Autodesk Fusion 360 part; units mm, degrees
(part 3 of 14)
  line L362 (718.6407, 200.025) -> (707.6422, 200.025)
  line L363 (707.6422, 200.025) -> (702.1429, 190.5)
  line L364 (702.1429, 190.5) -> (707.6422, 180.975)
  line L365 (707.6422, 180.975) -> (718.6407, 180.975)
  line L366 (724.1399, 190.5) -> (718.6407, 200.025)
  line L367 (718.6407, 180.975) -> (724.1399, 190.5)
  line L368 (737.8881, 211.1375) -> (726.8896, 211.1375)
  line L369 (726.8896, 211.1375) -> (721.3903, 201.6125)
  line L370 (721.3903, 201.6125) -> (726.8896, 192.0875)
  line L371 (726.8896, 192.0875) -> (737.8881, 192.0875)
  line L372 (743.3874, 201.6125) -> (737.8881, 211.1375)
  line L373 (737.8881, 192.0875) -> (743.3874, 201.6125)
  line L374 (757.1355, 222.25) -> (746.137, 222.25)
  line L375 (746.137, 222.25) -> (740.6377, 212.725)
  line L376 (740.6377, 212.725) -> (746.137, 203.2)
  line L377 (746.137, 203.2) -> (757.1355, 203.2)
  line L378 (762.6348, 212.725) -> (757.1355, 222.25)
  line L379 (757.1355, 203.2) -> (762.6348, 212.725)
  line L380 (-397.7094, -422.275) -> (-408.7079, -422.275)
  line L381 (-408.7079, -422.275) -> (-414.2072, -431.8)
  line L382 (-414.2072, -431.8) -> (-408.7079, -441.325)
  line L383 (-408.7079, -441.325) -> (-397.7094, -441.325)
  line L384 (-392.2101, -431.8) -> (-397.7094, -422.275)
  line L385 (-397.7094, -441.325) -> (-392.2101, -431.8)
  line L386 (-378.462, -411.1625) -> (-389.4605, -411.1625)
  line L387 (-389.4605, -411.1625) -> (-394.9597, -420.6875)
  line L388 (-394.9597, -420.6875) -> (-389.4605, -430.2125)
  line L389 (-389.4605, -430.2125) -> (-378.462, -430.2125)
  line L390 (-372.9627, -420.6875) -> (-378.462, -411.1625)
  line L391 (-378.462, -430.2125) -> (-372.9627, -420.6875)
  line L392 (-359.2145, -400.05) -> (-370.2131, -400.05)
  line L393 (-370.2131, -400.05) -> (-375.7123, -409.575)
  line L394 (-375.7123, -409.575) -> (-370.2131, -419.1)
  line L395 (-370.2131, -419.1) -> (-359.2145, -419.1)
  line L396 (-353.7153, -409.575) -> (-359.2145, -400.05)
  line L397 (-359.2145, -419.1) -> (-353.7153, -409.575)
  line L398 (-339.9671, -388.9375) -> (-350.9657, -388.9375)
  line L399 (-350.9657, -388.9375) -> (-356.4649, -398.4625)
  line L400 (-356.4649, -398.4625) -> (-350.9657, -407.9875)
  line L401 (-350.9657, -407.9875) -> (-339.9671, -407.9875)
  line L402 (-334.4679, -398.4625) -> (-339.9671, -388.9375)
  line L403 (-339.9671, -407.9875) -> (-334.4679, -398.4625)
  line L404 (-320.7197, -377.825) -> (-331.7182, -377.825)
  line L405 (-331.7182, -377.825) -> (-337.2175, -387.35)
  line L406 (-337.2175, -387.35) -> (-331.7182, -396.875)
  line L407 (-331.7182, -396.875) -> (-320.7197, -396.875)
  line L408 (-315.2205, -387.35) -> (-320.7197, -377.825)
  line L409 (-320.7197, -396.875) -> (-315.2205, -387.35)
  line L410 (-301.4723, -366.7125) -> (-312.4708, -366.7125)
  line L411 (-312.4708, -366.7125) -> (-317.9701, -376.2375)
  line L412 (-317.9701, -376.2375) -> (-312.4708, -385.7625)
  line L413 (-312.4708, -385.7625) -> (-301.4723, -385.7625)
  line L414 (-295.973, -376.2375) -> (-301.4723, -366.7125)
  line L415 (-301.4723, -385.7625) -> (-295.973, -376.2375)
  line L416 (-282.2249, -355.6) -> (-293.2234, -355.6)
  line L417 (-293.2234, -355.6) -> (-298.7227, -365.125)
  line L418 (-298.7227, -365.125) -> (-293.2234, -374.65)
  line L419 (-293.2234, -374.65) -> (-282.2249, -374.65)
  line L420 (-276.7256, -365.125) -> (-282.2249, -355.6)
  line L421 (-282.2249, -374.65) -> (-276.7256, -365.125)
  line L422 (-262.9775, -344.4875) -> (-273.976, -344.4875)
  line L423 (-273.976, -344.4875) -> (-279.4753, -354.0125)
  line L424 (-279.4753, -354.0125) -> (-273.976, -363.5375)
  line L425 (-273.976, -363.5375) -> (-262.9775, -363.5375)
  line L426 (-257.4782, -354.0125) -> (-262.9775, -344.4875)
  line L427 (-262.9775, -363.5375) -> (-257.4782, -354.0125)
  line L428 (-243.7301, -333.375) -> (-254.7286, -333.375)
  line L429 (-254.7286, -333.375) -> (-260.2278, -342.9)
  line L430 (-260.2278, -342.9) -> (-254.7286, -352.425)
  line L431 (-254.7286, -352.425) -> (-243.7301, -352.425)
  line L432 (-238.2308, -342.9) -> (-243.7301, -333.375)
  line L433 (-243.7301, -352.425) -> (-238.2308, -342.9)
  line L434 (-224.4826, -322.2625) -> (-235.4812, -322.2625)
  line L435 (-235.4812, -322.2625) -> (-240.9804, -331.7875)
  line L436 (-240.9804, -331.7875) -> (-235.4812, -341.3125)
  line L437 (-235.4812, -341.3125) -> (-224.4826, -341.3125)
  line L438 (-218.9834, -331.7875) -> (-224.4826, -322.2625)
  line L439 (-224.4826, -341.3125) -> (-218.9834, -331.7875)
  line L440 (-205.2352, -311.15) -> (-216.2337, -311.15)
  line L441 (-216.2337, -311.15) -> (-221.733, -320.675)
  line L442 (-221.733, -320.675) -> (-216.2337, -330.2)
  line L443 (-216.2337, -330.2) -> (-205.2352, -330.2)
  line L444 (-199.736, -320.675) -> (-205.2352, -311.15)
  line L445 (-205.2352, -330.2) -> (-199.736, -320.675)
  line L446 (-185.9878, -300.0375) -> (-196.9863, -300.0375)
  line L447 (-196.9863, -300.0375) -> (-202.4856, -309.5625)
  line L448 (-202.4856, -309.5625) -> (-196.9863, -319.0875)
  line L449 (-196.9863, -319.0875) -> (-185.9878, -319.0875)
  line L450 (-180.4886, -309.5625) -> (-185.9878, -300.0375)
  line L451 (-185.9878, -319.0875) -> (-180.4886, -309.5625)
  line L452 (-166.7404, -288.925) -> (-177.7389, -288.925)
  line L453 (-177.7389, -288.925) -> (-183.2382, -298.45)
  line L454 (-183.2382, -298.45) -> (-177.7389, -307.975)
  line L455 (-177.7389, -307.975) -> (-166.7404, -307.975)
  line L456 (-161.2411, -298.45) -> (-166.7404, -288.925)
  line L457 (-166.7404, -307.975) -> (-161.2411, -298.45)
  line L458 (-147.493, -277.8125) -> (-158.4915, -277.8125)
  line L459 (-158.4915, -277.8125) -> (-163.9908, -287.3375)
  line L460 (-163.9908, -287.3375) -> (-158.4915, -296.8625)
  line L461 (-158.4915, -296.8625) -> (-147.493, -296.8625)
  line L462 (-141.9937, -287.3375) -> (-147.493, -277.8125)
  line L463 (-147.493, -296.8625) -> (-141.9937, -287.3375)
  line L464 (-128.2456, -266.7) -> (-139.2441, -266.7)
  line L465 (-139.2441, -266.7) -> (-144.7434, -276.225)
  line L466 (-144.7434, -276.225) -> (-139.2441, -285.75)
  line L467 (-139.2441, -285.75) -> (-128.2456, -285.75)
  line L468 (-122.7463, -276.225) -> (-128.2456, -266.7)
  line L469 (-128.2456, -285.75) -> (-122.7463, -276.225)
  line L470 (-108.9982, -255.5875) -> (-119.9967, -255.5875)
  line L471 (-119.9967, -255.5875) -> (-125.4959, -265.1125)
  line L472 (-125.4959, -265.1125) -> (-119.9967, -274.6375)
  line L473 (-119.9967, -274.6375) -> (-108.9982, -274.6375)
  line L474 (-103.4989, -265.1125) -> (-108.9982, -255.5875)
  line L475 (-108.9982, -274.6375) -> (-103.4989, -265.1125)
  line L476 (-89.7507, -244.475) -> (-100.7493, -244.475)
  line L477 (-100.7493, -244.475) -> (-106.2485, -254)
  line L478 (-106.2485, -254) -> (-100.7493, -263.525)
  line L479 (-100.7493, -263.525) -> (-89.7507, -263.525)
  line L480 (-84.2515, -254) -> (-89.7507, -244.475)
  line L481 (-89.7507, -263.525) -> (-84.2515, -254)
  line L482 (-70.5033, -233.3625) -> (-81.5018, -233.3625)
  line L483 (-81.5018, -233.3625) -> (-87.0011, -242.8875)
  line L484 (-87.0011, -242.8875) -> (-81.5018, -252.4125)
  line L485 (-81.5018, -252.4125) -> (-70.5033, -252.4125)
  line L486 (-65.0041, -242.8875) -> (-70.5033, -233.3625)
  line L487 (-70.5033, -252.4125) -> (-65.0041, -242.8875)
  line L488 (-51.2559, -222.25) -> (-62.2544, -222.25)
  line L489 (-62.2544, -222.25) -> (-67.7537, -231.775)
  line L490 (-67.7537, -231.775) -> (-62.2544, -241.3)
  line L491 (-62.2544, -241.3) -> (-51.2559, -241.3)
  line L492 (-45.7566, -231.775) -> (-51.2559, -222.25)
  line L493 (-51.2559, -241.3) -> (-45.7566, -231.775)
  line L494 (-32.0085, -211.1375) -> (-43.007, -211.1375)
  line L495 (-43.007, -211.1375) -> (-48.5063, -220.6625)
  line L496 (-48.5063, -220.6625) -> (-43.007, -230.1875)
  line L497 (-43.007, -230.1875) -> (-32.0085, -230.1875)
  line L498 (-26.5092, -220.6625) -> (-32.0085, -211.1375)
  line L499 (-32.0085, -230.1875) -> (-26.5092, -220.6625)
  line L500 (-12.7611, -200.025) -> (-23.7596, -200.025)
  line L501 (-23.7596, -200.025) -> (-29.2589, -209.55)
  line L502 (-29.2589, -209.55) -> (-23.7596, -219.075)
  line L503 (-23.7596, -219.075) -> (-12.7611, -219.075)
  line L504 (-7.2618, -209.55) -> (-12.7611, -200.025)
  line L505 (-12.7611, -219.075) -> (-7.2618, -209.55)
  line L506 (6.4863, -188.9125) -> (-4.5122, -188.9125)
  line L507 (-4.5122, -188.9125) -> (-10.0114, -198.4375)
  line L508 (-10.0114, -198.4375) -> (-4.5122, -207.9625)
  line L509 (-4.5122, -207.9625) -> (6.4863, -207.9625)
  line L510 (11.9856, -198.4375) -> (6.4863, -188.9125)
  line L511 (6.4863, -207.9625) -> (11.9856, -198.4375)
  line L512 (25.7337, -177.8) -> (14.7352, -177.8)
  line L513 (14.7352, -177.8) -> (9.236, -187.325)
  line L514 (9.236, -187.325) -> (14.7352, -196.85)
  line L515 (14.7352, -196.85) -> (25.7337, -196.85)
  line L516 (31.233, -187.325) -> (25.7337, -177.8)
  line L517 (25.7337, -196.85) -> (31.233, -187.325)
  line L518 (44.9812, -166.6875) -> (33.9826, -166.6875)
  line L519 (33.9826, -166.6875) -> (28.4834, -176.2125)
  line L520 (28.4834, -176.2125) -> (33.9826, -185.7375)
  line L521 (33.9826, -185.7375) -> (44.9812, -185.7375)
  line L522 (50.4804, -176.2125) -> (44.9812, -166.6875)
  line L523 (44.9812, -185.7375) -> (50.4804, -176.2125)
  line L524 (64.2286, -155.575) -> (53.2301, -155.575)
  line L525 (53.2301, -155.575) -> (47.7308, -165.1)
  line L526 (47.7308, -165.1) -> (53.2301, -174.625)
  line L527 (53.2301, -174.625) -> (64.2286, -174.625)
  line L528 (69.7278, -165.1) -> (64.2286, -155.575)
  line L529 (64.2286, -174.625) -> (69.7278, -165.1)
  line L530 (83.476, -144.4625) -> (72.4775, -144.4625)
  line L531 (72.4775, -144.4625) -> (66.9782, -153.9875)
  line L532 (66.9782, -153.9875) -> (72.4775, -163.5125)
  line L533 (72.4775, -163.5125) -> (83.476, -163.5125)
  line L534 (88.9753, -153.9875) -> (83.476, -144.4625)
  line L535 (83.476, -163.5125) -> (88.9753, -153.9875)
  line L536 (102.7234, -133.35) -> (91.7249, -133.35)
  line L537 (91.7249, -133.35) -> (86.2256, -142.875)
  line L538 (86.2256, -142.875) -> (91.7249, -152.4)
  line L539 (91.7249, -152.4) -> (102.7234, -152.4)
  line L540 (108.2227, -142.875) -> (102.7234, -133.35)
  line L541 (102.7234, -152.4) -> (108.2227, -142.875)
  line L542 (121.9708, -122.2375) -> (110.9723, -122.2375)
  line L543 (110.9723, -122.2375) -> (105.473, -131.7625)
  line L544 (105.473, -131.7625) -> (110.9723, -141.2875)
  line L545 (110.9723, -141.2875) -> (121.9708, -141.2875)
  line L546 (127.4701, -131.7625) -> (121.9708, -122.2375)
  line L547 (121.9708, -141.2875) -> (127.4701, -131.7625)
  line L548 (141.2182, -111.125) -> (130.2197, -111.125)
  line L549 (130.2197, -111.125) -> (124.7205, -120.65)
  line L550 (124.7205, -120.65) -> (130.2197, -130.175)
  line L551 (130.2197, -130.175) -> (141.2182, -130.175)
  line L552 (146.7175, -120.65) -> (141.2182, -111.125)
  line L553 (141.2182, -130.175) -> (146.7175, -120.65)
  line L554 (160.4657, -100.0125) -> (149.4671, -100.0125)
  line L555 (149.4671, -100.0125) -> (143.9679, -109.5375)
  line L556 (143.9679, -109.5375) -> (149.4671, -119.0625)
  line L557 (149.4671, -119.0625) -> (160.4657, -119.0625)
  line L558 (165.9649, -109.5375) -> (160.4657, -100.0125)
  line L559 (160.4657, -119.0625) -> (165.9649, -109.5375)
  line L560 (179.7131, -88.9) -> (168.7145, -88.9)
  line L561 (168.7145, -88.9) -> (163.2153, -98.425)
  line L562 (163.2153, -98.425) -> (168.7145, -107.95)
  line L563 (168.7145, -107.95) -> (179.7131, -107.95)
  line L564 (185.2123, -98.425) -> (179.7131, -88.9)
  line L565 (179.7131, -107.95) -> (185.2123, -98.425)
  line L566 (198.9605, -77.7875) -> (187.962, -77.7875)
  line L567 (187.962, -77.7875) -> (182.4627, -87.3125)
  line L568 (182.4627, -87.3125) -> (187.962, -96.8375)
  line L569 (187.962, -96.8375) -> (198.9605, -96.8375)
  line L570 (204.4597, -87.3125) -> (198.9605, -77.7875)
  line L571 (198.9605, -96.8375) -> (204.4597, -87.3125)
  line L572 (218.2079, -66.675) -> (207.2094, -66.675)
  line L573 (207.2094, -66.675) -> (201.7101, -76.2)
  line L574 (201.7101, -76.2) -> (207.2094, -85.725)
  line L575 (207.2094, -85.725) -> (218.2079, -85.725)
  line L576 (223.7072, -76.2) -> (218.2079, -66.675)
  line L577 (218.2079, -85.725) -> (223.7072, -76.2)
  line L578 (237.4553, -55.5625) -> (226.4568, -55.5625)
  line L579 (226.4568, -55.5625) -> (220.9575, -65.0875)
  line L580 (220.9575, -65.0875) -> (226.4568, -74.6125)
  line L581 (226.4568, -74.6125) -> (237.4553, -74.6125)
  line L582 (242.9546, -65.0875) -> (237.4553, -55.5625)
  line L583 (237.4553, -74.6125) -> (242.9546, -65.0875)
  line L584 (256.7027, -44.45) -> (245.7042, -44.45)
  line L585 (245.7042, -44.45) -> (240.2049, -53.975)
  line L586 (240.2049, -53.975) -> (245.7042, -63.5)
  line L587 (245.7042, -63.5) -> (256.7027, -63.5)
  line L588 (262.202, -53.975) -> (256.7027, -44.45)
  line L589 (256.7027, -63.5) -> (262.202, -53.975)
  line L590 (275.9501, -33.3375) -> (264.9516, -33.3375)
  line L591 (264.9516, -33.3375) -> (259.4524, -42.8625)
  line L592 (259.4524, -42.8625) -> (264.9516, -52.3875)
  line L593 (264.9516, -52.3875) -> (275.9501, -52.3875)
  line L594 (281.4494, -42.8625) -> (275.9501, -33.3375)
  line L595 (275.9501, -52.3875) -> (281.4494, -42.8625)
  line L596 (295.1976, -22.225) -> (284.199, -22.225)
  line L597 (284.199, -22.225) -> (278.6998, -31.75)
  line L598 (278.6998, -31.75) -> (284.199, -41.275)
  line L599 (284.199, -41.275) -> (295.1976, -41.275)
  line L600 (300.6968, -31.75) -> (295.1976, -22.225)
  line L601 (295.1976, -41.275) -> (300.6968, -31.75)
  line L602 (314.445, -11.1125) -> (303.4464, -11.1125)
  line L603 (303.4464, -11.1125) -> (297.9472, -20.6375)
  line L604 (297.9472, -20.6375) -> (303.4464, -30.1625)
  line L605 (303.4464, -30.1625) -> (314.445, -30.1625)
  line L606 (319.9442, -20.6375) -> (314.445, -11.1125)
  line L607 (314.445, -30.1625) -> (319.9442, -20.6375)
  line L608 (333.6924, 0) -> (322.6939, 0)
  line L609 (322.6939, 0) -> (317.1946, -9.525)
  line L610 (317.1946, -9.525) -> (322.6939, -19.05)
  line L611 (322.6939, -19.05) -> (333.6924, -19.05)
  line L612 (339.1916, -9.525) -> (333.6924, 0)
  line L613 (333.6924, -19.05) -> (339.1916, -9.525)
  line L614 (352.9398, 11.1125) -> (341.9413, 11.1125)
  line L615 (341.9413, 11.1125) -> (336.442, 1.5875)
  line L616 (336.442, 1.5875) -> (341.9413, -7.9375)
  line L617 (341.9413, -7.9375) -> (352.9398, -7.9375)
  line L618 (358.4391, 1.5875) -> (352.9398, 11.1125)
  line L619 (352.9398, -7.9375) -> (358.4391, 1.5875)
  line L620 (372.1872, 22.225) -> (361.1887, 22.225)
  line L621 (361.1887, 22.225) -> (355.6894, 12.7)
  line L622 (355.6894, 12.7) -> (361.1887, 3.175)
  line L623 (361.1887, 3.175) -> (372.1872, 3.175)
  line L624 (377.6865, 12.7) -> (372.1872, 22.225)
  line L625 (372.1872, 3.175) -> (377.6865, 12.7)
  line L626 (391.4346, 33.3375) -> (380.4361, 33.3375)
  line L627 (380.4361, 33.3375) -> (374.9368, 23.8125)
  line L628 (374.9368, 23.8125) -> (380.4361, 14.2875)
  line L629 (380.4361, 14.2875) -> (391.4346, 14.2875)
  line L630 (396.9339, 23.8125) -> (391.4346, 33.3375)
  line L631 (391.4346, 14.2875) -> (396.9339, 23.8125)
  line L632 (410.682, 44.45) -> (399.6835, 44.45)
  line L633 (399.6835, 44.45) -> (394.1843, 34.925)
  line L634 (394.1843, 34.925) -> (399.6835, 25.4)
  line L635 (399.6835, 25.4) -> (410.682, 25.4)
  line L636 (416.1813, 34.925) -> (410.682, 44.45)
  line L637 (410.682, 25.4) -> (416.1813, 34.925)
  line L638 (429.9295, 55.5625) -> (418.9309, 55.5625)
  line L639 (418.9309, 55.5625) -> (413.4317, 46.0375)
  line L640 (413.4317, 46.0375) -> (418.9309, 36.5125)
  line L641 (418.9309, 36.5125) -> (429.9295, 36.5125)
  line L642 (435.4287, 46.0375) -> (429.9295, 55.5625)
  line L643 (429.9295, 36.5125) -> (435.4287, 46.0375)
  line L644 (449.1769, 66.675) -> (438.1783, 66.675)
  line L645 (438.1783, 66.675) -> (432.6791, 57.15)
  line L646 (432.6791, 57.15) -> (438.1783, 47.625)
  line L647 (438.1783, 47.625) -> (449.1769, 47.625)
  line L648 (454.6761, 57.15) -> (449.1769, 66.675)
  line L649 (449.1769, 47.625) -> (454.6761, 57.15)
  line L650 (468.4243, 77.7875) -> (457.4258, 77.7875)
  line L651 (457.4258, 77.7875) -> (451.9265, 68.2625)
  line L652 (451.9265, 68.2625) -> (457.4258, 58.7375)
  line L653 (457.4258, 58.7375) -> (468.4243, 58.7375)
  line L654 (473.9235, 68.2625) -> (468.4243, 77.7875)
  line L655 (468.4243, 58.7375) -> (473.9235, 68.2625)
  line L656 (487.6717, 88.9) -> (476.6732, 88.9)
  line L657 (476.6732, 88.9) -> (471.1739, 79.375)
  line L658 (471.1739, 79.375) -> (476.6732, 69.85)
  line L659 (476.6732, 69.85) -> (487.6717, 69.85)
  line L660 (493.171, 79.375) -> (487.6717, 88.9)
  line L661 (487.6717, 69.85) -> (493.171, 79.375)
  line L662 (506.9191, 100.0125) -> (495.9206, 100.0125)
  line L663 (495.9206, 100.0125) -> (490.4213, 90.4875)
  line L664 (490.4213, 90.4875) -> (495.9206, 80.9625)
  line L665 (495.9206, 80.9625) -> (506.9191, 80.9625)
  line L666 (512.4184, 90.4875) -> (506.9191, 100.0125)
  line L667 (506.9191, 80.9625) -> (512.4184, 90.4875)
  line L668 (526.1665, 111.125) -> (515.168, 111.125)
  line L669 (515.168, 111.125) -> (509.6687, 101.6)
  line L670 (509.6687, 101.6) -> (515.168, 92.075)
  line L671 (515.168, 92.075) -> (526.1665, 92.075)
  line L672 (531.6658, 101.6) -> (526.1665, 111.125)
  line L673 (526.1665, 92.075) -> (531.6658, 101.6)
  line L674 (545.4139, 122.2375) -> (534.4154, 122.2375)
  line L675 (534.4154, 122.2375) -> (528.9162, 112.7125)
  line L676 (528.9162, 112.7125) -> (534.4154, 103.1875)
  line L677 (534.4154, 103.1875) -> (545.4139, 103.1875)
  line L678 (550.9132, 112.7125) -> (545.4139, 122.2375)
  line L679 (545.4139, 103.1875) -> (550.9132, 112.7125)
  line L680 (564.6614, 133.35) -> (553.6628, 133.35)
  line L681 (553.6628, 133.35) -> (548.1636, 123.825)
  line L682 (548.1636, 123.825) -> (553.6628, 114.3)
  line L683 (553.6628, 114.3) -> (564.6614, 114.3)
  line L684 (570.1606, 123.825) -> (564.6614, 133.35)
  line L685 (564.6614, 114.3) -> (570.1606, 123.825)
  line L686 (583.9088, 144.4625) -> (572.9102, 144.4625)
  line L687 (572.9102, 144.4625) -> (567.411, 134.9375)
  line L688 (567.411, 134.9375) -> (572.9102, 125.4125)
  line L689 (572.9102, 125.4125) -> (583.9088, 125.4125)
  line L690 (589.408, 134.9375) -> (583.9088, 144.4625)
  line L691 (583.9088, 125.4125) -> (589.408, 134.9375)
  line L692 (603.1562, 155.575) -> (592.1577, 155.575)
  line L693 (592.1577, 155.575) -> (586.6584, 146.05)
  line L694 (586.6584, 146.05) -> (592.1577, 136.525)
  line L695 (592.1577, 136.525) -> (603.1562, 136.525)
  line L696 (608.6554, 146.05) -> (603.1562, 155.575)
  line L697 (603.1562, 136.525) -> (608.6554, 146.05)
  line L698 (622.4036, 166.6875) -> (611.4051, 166.6875)
  line L699 (611.4051, 166.6875) -> (605.9058, 157.1625)
  line L700 (605.9058, 157.1625) -> (611.4051, 147.6375)
  line L701 (611.4051, 147.6375) -> (622.4036, 147.6375)
  line L702 (627.9029, 157.1625) -> (622.4036, 166.6875)
  line L703 (622.4036, 147.6375) -> (627.9029, 157.1625)
  line L704 (641.651, 177.8) -> (630.6525, 177.8)
  line L705 (630.6525, 177.8) -> (625.1532, 168.275)
  line L706 (625.1532, 168.275) -> (630.6525, 158.75)
  line L707 (630.6525, 158.75) -> (641.651, 158.75)
  line L708 (647.1503, 168.275) -> (641.651, 177.8)
  line L709 (641.651, 158.75) -> (647.1503, 168.275)
  line L710 (660.8984, 188.9125) -> (649.8999, 188.9125)
  line L711 (649.8999, 188.9125) -> (644.4006, 179.3875)
  line L712 (644.4006, 179.3875) -> (649.8999, 169.8625)
  line L713 (649.8999, 169.8625) -> (660.8984, 169.8625)
  line L714 (666.3977, 179.3875) -> (660.8984, 188.9125)
  line L715 (660.8984, 169.8625) -> (666.3977, 179.3875)
  line L716 (680.1458, 200.025) -> (669.1473, 200.025)
  line L717 (669.1473, 200.025) -> (663.6481, 190.5)
  line L718 (663.6481, 190.5) -> (669.1473, 180.975)
  line L719 (669.1473, 180.975) -> (680.1458, 180.975)
  line L720 (685.6451, 190.5) -> (680.1458, 200.025)
  line L721 (680.1458, 180.975) -> (685.6451, 190.5)
  line L722 (699.3933, 211.1375) -> (688.3947, 211.1375)
  line L723 (688.3947, 211.1375) -> (682.8955, 201.6125)
  line L724 (682.8955, 201.6125) -> (688.3947, 192.0875)
  line L725 (688.3947, 192.0875) -> (699.3933, 192.0875)
  line L726 (704.8925, 201.6125) -> (699.3933, 211.1375)
  line L727 (699.3933, 192.0875) -> (704.8925, 201.6125)
  line L728 (718.6407, 222.25) -> (707.6422, 222.25)
  line L729 (707.6422, 222.25) -> (702.1429, 212.725)
  line L730 (702.1429, 212.725) -> (707.6422, 203.2)
  line L731 (707.6422, 203.2) -> (718.6407, 203.2)
  line L732 (724.1399, 212.725) -> (718.6407, 222.25)
  line L733 (718.6407, 203.2) -> (724.1399, 212.725)
  line L734 (737.8881, 233.3625) -> (726.8896, 233.3625)
  line L735 (726.8896, 233.3625) -> (721.3903, 223.8375)
  line L736 (721.3903, 223.8375) -> (726.8896, 214.3125)
  line L737 (726.8896, 214.3125) -> (737.8881, 214.3125)
  line L738 (743.3874, 223.8375) -> (737.8881, 233.3625)
  line L739 (737.8881, 214.3125) -> (743.3874, 223.8375)
  line L740 (-416.9568, -411.1625) -> (-427.9553, -411.1625)
  line L741 (-427.9553, -411.1625) -> (-433.4546, -420.6875)
  line L742 (-433.4546, -420.6875) -> (-427.9553, -430.2125)
  line L743 (-427.9553, -430.2125) -> (-416.9568, -430.2125)
  line L744 (-411.4575, -420.6875) -> (-416.9568, -411.1625)
  line L745 (-416.9568, -430.2125) -> (-411.4575, -420.6875)
  line L746 (-397.7094, -400.05) -> (-408.7079, -400.05)
  line L747 (-408.7079, -400.05) -> (-414.2072, -409.575)
  line L748 (-414.2072, -409.575) -> (-408.7079, -419.1)
  line L749 (-408.7079, -419.1) -> (-397.7094, -419.1)
  line L750 (-392.2101, -409.575) -> (-397.7094, -400.05)
  line L751 (-397.7094, -419.1) -> (-392.2101, -409.575)
  line L752 (-378.462, -388.9375) -> (-389.4605, -388.9375)
  line L753 (-389.4605, -388.9375) -> (-394.9597, -398.4625)
  line L754 (-394.9597, -398.4625) -> (-389.4605, -407.9875)
  line L755 (-389.4605, -407.9875) -> (-378.462, -407.9875)
  line L756 (-372.9627, -398.4625) -> (-378.462, -388.9375)
  line L757 (-378.462, -407.9875) -> (-372.9627, -398.4625)
  line L758 (-359.2145, -377.825) -> (-370.2131, -377.825)
  line L759 (-370.2131, -377.825) -> (-375.7123, -387.35)
  line L760 (-375.7123, -387.35) -> (-370.2131, -396.875)
  line L761 (-370.2131, -396.875) -> (-359.2145, -396.875)
  line L762 (-353.7153, -387.35) -> (-359.2145, -377.825)
  line L763 (-359.2145, -396.875) -> (-353.7153, -387.35)
  line L764 (-339.9671, -366.7125) -> (-350.9657, -366.7125)
  line L765 (-350.9657, -366.7125) -> (-356.4649, -376.2375)
  line L766 (-356.4649, -376.2375) -> (-350.9657, -385.7625)
  line L767 (-350.9657, -385.7625) -> (-339.9671, -385.7625)
  line L768 (-334.4679, -376.2375) -> (-339.9671, -366.7125)
  line L769 (-339.9671, -385.7625) -> (-334.4679, -376.2375)
  line L770 (-320.7197, -355.6) -> (-331.7182, -355.6)
  line L771 (-331.7182, -355.6) -> (-337.2175, -365.125)
  line L772 (-337.2175, -365.125) -> (-331.7182, -374.65)
  line L773 (-331.7182, -374.65) -> (-320.7197, -374.65)
  line L774 (-315.2205, -365.125) -> (-320.7197, -355.6)
  line L775 (-320.7197, -374.65) -> (-315.2205, -365.125)
  line L776 (-301.4723, -344.4875) -> (-312.4708, -344.4875)
  line L777 (-312.4708, -344.4875) -> (-317.9701, -354.0125)
  line L778 (-317.9701, -354.0125) -> (-312.4708, -363.5375)
  line L779 (-312.4708, -363.5375) -> (-301.4723, -363.5375)
  line L780 (-295.973, -354.0125) -> (-301.4723, -344.4875)
  line L781 (-301.4723, -363.5375) -> (-295.973, -354.0125)
  line L782 (-282.2249, -333.375) -> (-293.2234, -333.375)
  line L783 (-293.2234, -333.375) -> (-298.7227, -342.9)
  line L784 (-298.7227, -342.9) -> (-293.2234, -352.425)
  line L785 (-293.2234, -352.425) -> (-282.2249, -352.425)
  line L786 (-276.7256, -342.9) -> (-282.2249, -333.375)
  line L787 (-282.2249, -352.425) -> (-276.7256, -342.9)
  line L788 (-262.9775, -322.2625) -> (-273.976, -322.2625)
  line L789 (-273.976, -322.2625) -> (-279.4753, -331.7875)
  line L790 (-279.4753, -331.7875) -> (-273.976, -341.3125)
  line L791 (-273.976, -341.3125) -> (-262.9775, -341.3125)
  line L792 (-257.4782, -331.7875) -> (-262.9775, -322.2625)
  line L793 (-262.9775, -341.3125) -> (-257.4782, -331.7875)
  line L794 (-243.7301, -311.15) -> (-254.7286, -311.15)
  line L795 (-254.7286, -311.15) -> (-260.2278, -320.675)
  line L796 (-260.2278, -320.675) -> (-254.7286, -330.2)
  line L797 (-254.7286, -330.2) -> (-243.7301, -330.2)
  line L798 (-238.2308, -320.675) -> (-243.7301, -311.15)
  line L799 (-243.7301, -330.2) -> (-238.2308, -320.675)
  line L800 (-224.4826, -300.0375) -> (-235.4812, -300.0375)
  line L801 (-235.4812, -300.0375) -> (-240.9804, -309.5625)
  line L802 (-240.9804, -309.5625) -> (-235.4812, -319.0875)
  line L803 (-235.4812, -319.0875) -> (-224.4826, -319.0875)
  line L804 (-218.9834, -309.5625) -> (-224.4826, -300.0375)
  line L805 (-224.4826, -319.0875) -> (-218.9834, -309.5625)
  line L806 (-205.2352, -288.925) -> (-216.2337, -288.925)
  line L807 (-216.2337, -288.925) -> (-221.733, -298.45)
  line L808 (-221.733, -298.45) -> (-216.2337, -307.975)
  line L809 (-216.2337, -307.975) -> (-205.2352, -307.975)
  line L810 (-199.736, -298.45) -> (-205.2352, -288.925)
  line L811 (-205.2352, -307.975) -> (-199.736, -298.45)
  line L812 (-185.9878, -277.8125) -> (-196.9863, -277.8125)
  line L813 (-196.9863, -277.8125) -> (-202.4856, -287.3375)
  line L814 (-202.4856, -287.3375) -> (-196.9863, -296.8625)
  line L815 (-196.9863, -296.8625) -> (-185.9878, -296.8625)
  line L816 (-180.4886, -287.3375) -> (-185.9878, -277.8125)
  line L817 (-185.9878, -296.8625) -> (-180.4886, -287.3375)
  line L818 (-166.7404, -266.7) -> (-177.7389, -266.7)
  line L819 (-177.7389, -266.7) -> (-183.2382, -276.225)
  line L820 (-183.2382, -276.225) -> (-177.7389, -285.75)
  line L821 (-177.7389, -285.75) -> (-166.7404, -285.75)
  line L822 (-161.2411, -276.225) -> (-166.7404, -266.7)
  line L823 (-166.7404, -285.75) -> (-161.2411, -276.225)
  line L824 (-147.493, -255.5875) -> (-158.4915, -255.5875)
  line L825 (-158.4915, -255.5875) -> (-163.9908, -265.1125)
  line L826 (-163.9908, -265.1125) -> (-158.4915, -274.6375)
  line L827 (-158.4915, -274.6375) -> (-147.493, -274.6375)
  line L828 (-141.9937, -265.1125) -> (-147.493, -255.5875)
  line L829 (-147.493, -274.6375) -> (-141.9937, -265.1125)
  line L830 (-128.2456, -244.475) -> (-139.2441, -244.475)
  line L831 (-139.2441, -244.475) -> (-144.7434, -254)
  line L832 (-144.7434, -254) -> (-139.2441, -263.525)
  line L833 (-139.2441, -263.525) -> (-128.2456, -263.525)
  line L834 (-122.7463, -254) -> (-128.2456, -244.475)
  line L835 (-128.2456, -263.525) -> (-122.7463, -254)
  line L836 (-108.9982, -233.3625) -> (-119.9967, -233.3625)
  line L837 (-119.9967, -233.3625) -> (-125.4959, -242.8875)
  line L838 (-125.4959, -242.8875) -> (-119.9967, -252.4125)
  line L839 (-119.9967, -252.4125) -> (-108.9982, -252.4125)
  line L840 (-103.4989, -242.8875) -> (-108.9982, -233.3625)
  line L841 (-108.9982, -252.4125) -> (-103.4989, -242.8875)
  line L842 (-89.7507, -222.25) -> (-100.7493, -222.25)
  line L843 (-100.7493, -222.25) -> (-106.2485, -231.775)
  line L844 (-106.2485, -231.775) -> (-100.7493, -241.3)
  line L845 (-100.7493, -241.3) -> (-89.7507, -241.3)
  line L846 (-84.2515, -231.775) -> (-89.7507, -222.25)
  line L847 (-89.7507, -241.3) -> (-84.2515, -231.775)
  line L848 (-70.5033, -211.1375) -> (-81.5018, -211.1375)
  line L849 (-81.5018, -211.1375) -> (-87.0011, -220.6625)
  line L850 (-87.0011, -220.6625) -> (-81.5018, -230.1875)
  line L851 (-81.5018, -230.1875) -> (-70.5033, -230.1875)
  line L852 (-65.0041, -220.6625) -> (-70.5033, -211.1375)
  line L853 (-70.5033, -230.1875) -> (-65.0041, -220.6625)
  line L854 (-51.2559, -200.025) -> (-62.2544, -200.025)
  line L855 (-62.2544, -200.025) -> (-67.7537, -209.55)
  line L856 (-67.7537, -209.55) -> (-62.2544, -219.075)
  line L857 (-62.2544, -219.075) -> (-51.2559, -219.075)
  line L858 (-45.7566, -209.55) -> (-51.2559, -200.025)
  line L859 (-51.2559, -219.075) -> (-45.7566, -209.55)
  line L860 (-32.0085, -188.9125) -> (-43.007, -188.9125)
  line L861 (-43.007, -188.9125) -> (-48.5063, -198.4375)
  line L862 (-48.5063, -198.4375) -> (-43.007, -207.9625)
  line L863 (-43.007, -207.9625) -> (-32.0085, -207.9625)
  line L864 (-26.5092, -198.4375) -> (-32.0085, -188.9125)
  line L865 (-32.0085, -207.9625) -> (-26.5092, -198.4375)
  line L866 (-12.7611, -177.8) -> (-23.7596, -177.8)
  line L867 (-23.7596, -177.8) -> (-29.2589, -187.325)
  line L868 (-29.2589, -187.325) -> (-23.7596, -196.85)
  line L869 (-23.7596, -196.85) -> (-12.7611, -196.85)
  line L870 (-7.2618, -187.325) -> (-12.7611, -177.8)
  line L871 (-12.7611, -196.85) -> (-7.2618, -187.325)
  line L872 (6.4863, -166.6875) -> (-4.5122, -166.6875)
  line L873 (-4.5122, -166.6875) -> (-10.0114, -176.2125)
  line L874 (-10.0114, -176.2125) -> (-4.5122, -185.7375)
  line L875 (-4.5122, -185.7375) -> (6.4863, -185.7375)
  line L876 (11.9856, -176.2125) -> (6.4863, -166.6875)
  line L877 (6.4863, -185.7375) -> (11.9856, -176.2125)
  line L878 (25.7337, -155.575) -> (14.7352, -155.575)
  line L879 (14.7352, -155.575) -> (9.236, -165.1)
  line L880 (9.236, -165.1) -> (14.7352, -174.625)
  line L881 (14.7352, -174.625) -> (25.7337, -174.625)
  line L882 (31.233, -165.1) -> (25.7337, -155.575)
  line L883 (25.7337, -174.625) -> (31.233, -165.1)
  line L884 (44.9812, -144.4625) -> (33.9826, -144.4625)
  line L885 (33.9826, -144.4625) -> (28.4834, -153.9875)
  line L886 (28.4834, -153.9875) -> (33.9826, -163.5125)
  line L887 (33.9826, -163.5125) -> (44.9812, -163.5125)
  line L888 (50.4804, -153.9875) -> (44.9812, -144.4625)
  line L889 (44.9812, -163.5125) -> (50.4804, -153.9875)
  line L890 (64.2286, -133.35) -> (53.2301, -133.35)
  line L891 (53.2301, -133.35) -> (47.7308, -142.875)
  line L892 (47.7308, -142.875) -> (53.2301, -152.4)
  line L893 (53.2301, -152.4) -> (64.2286, -152.4)
  line L894 (69.7278, -142.875) -> (64.2286, -133.35)
  line L895 (64.2286, -152.4) -> (69.7278, -142.875)
  line L896 (83.476, -122.2375) -> (72.4775, -122.2375)
  line L897 (72.4775, -122.2375) -> (66.9782, -131.7625)
  line L898 (66.9782, -131.7625) -> (72.4775, -141.2875)
  line L899 (72.4775, -141.2875) -> (83.476, -141.2875)
  line L900 (88.9753, -131.7625) -> (83.476, -122.2375)
  line L901 (83.476, -141.2875) -> (88.9753, -131.7625)
  line L902 (102.7234, -111.125) -> (91.7249, -111.125)
  line L903 (91.7249, -111.125) -> (86.2256, -120.65)
  line L904 (86.2256, -120.65) -> (91.7249, -130.175)
  line L905 (91.7249, -130.175) -> (102.7234, -130.175)
  line L906 (108.2227, -120.65) -> (102.7234, -111.125)
  line L907 (102.7234, -130.175) -> (108.2227, -120.65)
  line L908 (121.9708, -100.0125) -> (110.9723, -100.0125)
  line L909 (110.9723, -100.0125) -> (105.473, -109.5375)
  line L910 (105.473, -109.5375) -> (110.9723, -119.0625)
  line L911 (110.9723, -119.0625) -> (121.9708, -119.0625)
  line L912 (127.4701, -109.5375) -> (121.9708, -100.0125)
  line L913 (121.9708, -119.0625) -> (127.4701, -109.5375)
  line L914 (141.2182, -88.9) -> (130.2197, -88.9)
  line L915 (130.2197, -88.9) -> (124.7205, -98.425)
  line L916 (124.7205, -98.425) -> (130.2197, -107.95)
  line L917 (130.2197, -107.95) -> (141.2182, -107.95)
  line L918 (146.7175, -98.425) -> (141.2182, -88.9)
  line L919 (141.2182, -107.95) -> (146.7175, -98.425)
  line L920 (160.4657, -77.7875) -> (149.4671, -77.7875)
  line L921 (149.4671, -77.7875) -> (143.9679, -87.3125)
  line L922 (143.9679, -87.3125) -> (149.4671, -96.8375)
  line L923 (149.4671, -96.8375) -> (160.4657, -96.8375)
  line L924 (165.9649, -87.3125) -> (160.4657, -77.7875)
  line L925 (160.4657, -96.8375) -> (165.9649, -87.3125)
  line L926 (179.7131, -66.675) -> (168.7145, -66.675)
  line L927 (168.7145, -66.675) -> (163.2153, -76.2)
  line L928 (163.2153, -76.2) -> (168.7145, -85.725)
  line L929 (168.7145, -85.725) -> (179.7131, -85.725)
  line L930 (185.2123, -76.2) -> (179.7131, -66.675)
  line L931 (179.7131, -85.725) -> (185.2123, -76.2)
  line L932 (198.9605, -55.5625) -> (187.962, -55.5625)
  line L933 (187.962, -55.5625) -> (182.4627, -65.0875)
  line L934 (182.4627, -65.0875) -> (187.962, -74.6125)
  line L935 (187.962, -74.6125) -> (198.9605, -74.6125)
  line L936 (204.4597, -65.0875) -> (198.9605, -55.5625)
  line L937 (198.9605, -74.6125) -> (204.4597, -65.0875)
  line L938 (218.2079, -44.45) -> (207.2094, -44.45)
  line L939 (207.2094, -44.45) -> (201.7101, -53.975)
  line L940 (201.7101, -53.975) -> (207.2094, -63.5)
  line L941 (207.2094, -63.5) -> (218.2079, -63.5)
  line L942 (223.7072, -53.975) -> (218.2079, -44.45)
  line L943 (218.2079, -63.5) -> (223.7072, -53.975)
  line L944 (237.4553, -33.3375) -> (226.4568, -33.3375)
  line L945 (226.4568, -33.3375) -> (220.9575, -42.8625)
  line L946 (220.9575, -42.8625) -> (226.4568, -52.3875)
  line L947 (226.4568, -52.3875) -> (237.4553, -52.3875)
  line L948 (242.9546, -42.8625) -> (237.4553, -33.3375)
  line L949 (237.4553, -52.3875) -> (242.9546, -42.8625)
  line L950 (256.7027, -22.225) -> (245.7042, -22.225)
  line L951 (245.7042, -22.225) -> (240.2049, -31.75)
  line L952 (240.2049, -31.75) -> (245.7042, -41.275)
  line L953 (245.7042, -41.275) -> (256.7027, -41.275)
  line L954 (262.202, -31.75) -> (256.7027, -22.225)
  line L955 (256.7027, -41.275) -> (262.202, -31.75)
  line L956 (275.9501, -11.1125) -> (264.9516, -11.1125)
  line L957 (264.9516, -11.1125) -> (259.4524, -20.6375)
  line L958 (259.4524, -20.6375) -> (264.9516, -30.1625)
  line L959 (264.9516, -30.1625) -> (275.9501, -30.1625)
  line L960 (281.4494, -20.6375) -> (275.9501, -11.1125)
  line L961 (275.9501, -30.1625) -> (281.4494, -20.6375)
  line L962 (295.1976, 0) -> (284.199, 0)
  line L963 (284.199, 0) -> (278.6998, -9.525)
  line L964 (278.6998, -9.525) -> (284.199, -19.05)
  line L965 (284.199, -19.05) -> (295.1976, -19.05)
  line L966 (300.6968, -9.525) -> (295.1976, 0)
  line L967 (295.1976, -19.05) -> (300.6968, -9.525)
  line L968 (314.445, 11.1125) -> (303.4464, 11.1125)
  line L969 (303.4464, 11.1125) -> (297.9472, 1.5875)
  line L970 (297.9472, 1.5875) -> (303.4464, -7.9375)
  line L971 (303.4464, -7.9375) -> (314.445, -7.9375)
  line L972 (319.9442, 1.5875) -> (314.445, 11.1125)
  line L973 (314.445, -7.9375) -> (319.9442, 1.5875)
  line L974 (333.6924, 22.225) -> (322.6939, 22.225)
  line L975 (322.6939, 22.225) -> (317.1946, 12.7)
  line L976 (317.1946, 12.7) -> (322.6939, 3.175)
  line L977 (322.6939, 3.175) -> (333.6924, 3.175)
  line L978 (339.1916, 12.7) -> (333.6924, 22.225)
  line L979 (333.6924, 3.175) -> (339.1916, 12.7)
  line L980 (352.9398, 33.3375) -> (341.9413, 33.3375)
  line L981 (341.9413, 33.3375) -> (336.442, 23.8125)
  line L982 (336.442, 23.8125) -> (341.9413, 14.2875)
  line L983 (341.9413, 14.2875) -> (352.9398, 14.2875)
  line L984 (358.4391, 23.8125) -> (352.9398, 33.3375)
  line L985 (352.9398, 14.2875) -> (358.4391, 23.8125)
  line L986 (372.1872, 44.45) -> (361.1887, 44.45)
  line L987 (361.1887, 44.45) -> (355.6894, 34.925)
  line L988 (355.6894, 34.925) -> (361.1887, 25.4)
  line L989 (361.1887, 25.4) -> (372.1872, 25.4)
  line L990 (377.6865, 34.925) -> (372.1872, 44.45)
  line L991 (372.1872, 25.4) -> (377.6865, 34.925)
  line L992 (391.4346, 55.5625) -> (380.4361, 55.5625)
  line L993 (380.4361, 55.5625) -> (374.9368, 46.0375)
  line L994 (374.9368, 46.0375) -> (380.4361, 36.5125)
  line L995 (380.4361, 36.5125) -> (391.4346, 36.5125)
  line L996 (396.9339, 46.0375) -> (391.4346, 55.5625)
  line L997 (391.4346, 36.5125) -> (396.9339, 46.0375)
  line L998 (410.682, 66.675) -> (399.6835, 66.675)
  line L999 (399.6835, 66.675) -> (394.1843, 57.15)
  line L1000 (394.1843, 57.15) -> (399.6835, 47.625)
  line L1001 (399.6835, 47.625) -> (410.682, 47.625)
  line L1002 (416.1813, 57.15) -> (410.682, 66.675)
  line L1003 (410.682, 47.625) -> (416.1813, 57.15)
  line L1004 (429.9295, 77.7875) -> (418.9309, 77.7875)
  line L1005 (418.9309, 77.7875) -> (413.4317, 68.2625)
  line L1006 (413.4317, 68.2625) -> (418.9309, 58.7375)
  line L1007 (418.9309, 58.7375) -> (429.9295, 58.7375)
  line L1008 (435.4287, 68.2625) -> (429.9295, 77.7875)
  line L1009 (429.9295, 58.7375) -> (435.4287, 68.2625)
  line L1010 (449.1769, 88.9) -> (438.1783, 88.9)
  line L1011 (438.1783, 88.9) -> (432.6791, 79.375)
  line L1012 (432.6791, 79.375) -> (438.1783, 69.85)
  line L1013 (438.1783, 69.85) -> (449.1769, 69.85)
  line L1014 (454.6761, 79.375) -> (449.1769, 88.9)
  line L1015 (449.1769, 69.85) -> (454.6761, 79.375)
  line L1016 (468.4243, 100.0125) -> (457.4258, 100.0125)
  line L1017 (457.4258, 100.0125) -> (451.9265, 90.4875)
  line L1018 (451.9265, 90.4875) -> (457.4258, 80.9625)
  line L1019 (457.4258, 80.9625) -> (468.4243, 80.9625)
  line L1020 (473.9235, 90.4875) -> (468.4243, 100.0125)
  line L1021 (468.4243, 80.9625) -> (473.9235, 90.4875)
  line L1022 (487.6717, 111.125) -> (476.6732, 111.125)
  line L1023 (476.6732, 111.125) -> (471.1739, 101.6)
  line L1024 (471.1739, 101.6) -> (476.6732, 92.075)
  line L1025 (476.6732, 92.075) -> (487.6717, 92.075)
  line L1026 (493.171, 101.6) -> (487.6717, 111.125)
  line L1027 (487.6717, 92.075) -> (493.171, 101.6)
  line L1028 (506.9191, 122.2375) -> (495.9206, 122.2375)
  line L1029 (495.9206, 122.2375) -> (490.4213, 112.7125)
  line L1030 (490.4213, 112.7125) -> (495.9206, 103.1875)
  line L1031 (495.9206, 103.1875) -> (506.9191, 103.1875)
  line L1032 (512.4184, 112.7125) -> (506.9191, 122.2375)
  line L1033 (506.9191, 103.1875) -> (512.4184, 112.7125)
  line L1034 (526.1665, 133.35) -> (515.168, 133.35)
  line L1035 (515.168, 133.35) -> (509.6687, 123.825)
  line L1036 (509.6687, 123.825) -> (515.168, 114.3)
  line L1037 (515.168, 114.3) -> (526.1665, 114.3)
  line L1038 (531.6658, 123.825) -> (526.1665, 133.35)
  line L1039 (526.1665, 114.3) -> (531.6658, 123.825)
  line L1040 (545.4139, 144.4625) -> (534.4154, 144.4625)
  line L1041 (534.4154, 144.4625) -> (528.9162, 134.9375)
  line L1042 (528.9162, 134.9375) -> (534.4154, 125.4125)
  line L1043 (534.4154, 125.4125) -> (545.4139, 125.4125)
  line L1044 (550.9132, 134.9375) -> (545.4139, 144.4625)
  line L1045 (545.4139, 125.4125) -> (550.9132, 134.9375)
  line L1046 (564.6614, 155.575) -> (553.6628, 155.575)
  line L1047 (553.6628, 155.575) -> (548.1636, 146.05)
  line L1048 (548.1636, 146.05) -> (553.6628, 136.525)
  line L1049 (553.6628, 136.525) -> (564.6614, 136.525)
  line L1050 (570.1606, 146.05) -> (564.6614, 155.575)
  line L1051 (564.6614, 136.525) -> (570.1606, 146.05)
  line L1052 (583.9088, 166.6875) -> (572.9102, 166.6875)
  line L1053 (572.9102, 166.6875) -> (567.411, 157.1625)
  line L1054 (567.411, 157.1625) -> (572.9102, 147.6375)
  line L1055 (572.9102, 147.6375) -> (583.9088, 147.6375)
  line L1056 (589.408, 157.1625) -> (583.9088, 166.6875)
  line L1057 (583.9088, 147.6375) -> (589.408, 157.1625)
  line L1058 (603.1562, 177.8) -> (592.1577, 177.8)
  line L1059 (592.1577, 177.8) -> (586.6584, 168.275)
  line L1060 (586.6584, 168.275) -> (592.1577, 158.75)
  line L1061 (592.1577, 158.75) -> (603.1562, 158.75)
  line L1062 (608.6554, 168.275) -> (603.1562, 177.8)
  line L1063 (603.1562, 158.75) -> (608.6554, 168.275)
  line L1064 (622.4036, 188.9125) -> (611.4051, 188.9125)
  line L1065 (611.4051, 188.9125) -> (605.9058, 179.3875)
  line L1066 (605.9058, 179.3875) -> (611.4051, 169.8625)
  line L1067 (611.4051, 169.8625) -> (622.4036, 169.8625)
  line L1068 (627.9029, 179.3875) -> (622.4036, 188.9125)
  line L1069 (622.4036, 169.8625) -> (627.9029, 179.3875)
  line L1070 (641.651, 200.025) -> (630.6525, 200.025)
  line L1071 (630.6525, 200.025) -> (625.1532, 190.5)
  line L1072 (625.1532, 190.5) -> (630.6525, 180.975)
  line L1073 (630.6525, 180.975) -> (641.651, 180.975)
  line L1074 (647.1503, 190.5) -> (641.651, 200.025)
  line L1075 (641.651, 180.975) -> (647.1503, 190.5)
  line L1076 (660.8984, 211.1375) -> (649.8999, 211.1375)
  line L1077 (649.8999, 211.1375) -> (644.4006, 201.6125)
  line L1078 (644.4006, 201.6125) -> (649.8999, 192.0875)
  line L1079 (649.8999, 192.0875) -> (660.8984, 192.0875)
  line L1080 (666.3977, 201.6125) -> (660.8984, 211.1375)
  line L1081 (660.8984, 192.0875) -> (666.3977, 201.6125)
  line L1082 (680.1458, 222.25) -> (669.1473, 222.25)
  line L1083 (669.1473, 222.25) -> (663.6481, 212.725)
  line L1084 (663.6481, 212.725) -> (669.1473, 203.2)
  line L1085 (669.1473, 203.2) -> (680.1458, 203.2)
  line L1086 (685.6451, 212.725) -> (680.1458, 222.25)
  line L1087 (680.1458, 203.2) -> (685.6451, 212.725)
  line L1088 (699.3933, 233.3625) -> (688.3947, 233.3625)
  line L1089 (688.3947, 233.3625) -> (682.8955, 223.8375)
  line L1090 (682.8955, 223.8375) -> (688.3947, 214.3125)
  line L1091 (688.3947, 214.3125) -> (699.3933, 214.3125)
  line L1092 (704.8925, 223.8375) -> (699.3933, 233.3625)
  line L1093 (699.3933, 214.3125) -> (704.8925, 223.8375)
  line L1094 (718.6407, 244.475) -> (707.6422, 244.475)
  line L1095 (707.6422, 244.475) -> (702.1429, 234.95)
  line L1096 (702.1429, 234.95) -> (707.6422, 225.425)
  line L1097 (707.6422, 225.425) -> (718.6407, 225.425)
  line L1098 (724.1399, 234.95) -> (718.6407, 244.475)
  line L1099 (718.6407, 225.425) -> (724.1399, 234.95)
  line L1100 (-436.2042, -400.05) -> (-447.2027, -400.05)
  line L1101 (-447.2027, -400.05) -> (-452.702, -409.575)
  line L1102 (-452.702, -409.575) -> (-447.2027, -419.1)
  line L1103 (-447.2027, -419.1) -> (-436.2042, -419.1)
  line L1104 (-430.7049, -409.575) -> (-436.2042, -400.05)
  line L1105 (-436.2042, -419.1) -> (-430.7049, -409.575)
  line L1106 (-416.9568, -388.9375) -> (-427.9553, -388.9375)
  line L1107 (-427.9553, -388.9375) -> (-433.4546, -398.4625)
  line L1108 (-433.4546, -398.4625) -> (-427.9553, -407.9875)
  line L1109 (-427.9553, -407.9875) -> (-416.9568, -407.9875)
  line L1110 (-411.4575, -398.4625) -> (-416.9568, -388.9375)
  line L1111 (-416.9568, -407.9875) -> (-411.4575, -398.4625)
  line L1112 (-397.7094, -377.825) -> (-408.7079, -377.825)
  line L1113 (-408.7079, -377.825) -> (-414.2072, -387.35)
  line L1114 (-414.2072, -387.35) -> (-408.7079, -396.875)
  line L1115 (-408.7079, -396.875) -> (-397.7094, -396.875)
  line L1116 (-392.2101, -387.35) -> (-397.7094, -377.825)
  line L1117 (-397.7094, -396.875) -> (-392.2101, -387.35)
  line L1118 (-378.462, -366.7125) -> (-389.4605, -366.7125)
  line L1119 (-389.4605, -366.7125) -> (-394.9597, -376.2375)
  line L1120 (-394.9597, -376.2375) -> (-389.4605, -385.7625)
  line L1121 (-389.4605, -385.7625) -> (-378.462, -385.7625)
  line L1122 (-372.9627, -376.2375) -> (-378.462, -366.7125)
  line L1123 (-378.462, -385.7625) -> (-372.9627, -376.2375)
  line L1124 (-359.2145, -355.6) -> (-370.2131, -355.6)
  line L1125 (-370.2131, -355.6) -> (-375.7123, -365.125)
  line L1126 (-375.7123, -365.125) -> (-370.2131, -374.65)
  line L1127 (-370.2131, -374.65) -> (-359.2145, -374.65)
  line L1128 (-353.7153, -365.125) -> (-359.2145, -355.6)
  line L1129 (-359.2145, -374.65) -> (-353.7153, -365.125)
  line L1130 (-339.9671, -344.4875) -> (-350.9657, -344.4875)
  line L1131 (-350.9657, -344.4875) -> (-356.4649, -354.0125)
  line L1132 (-356.4649, -354.0125) -> (-350.9657, -363.5375)
  line L1133 (-350.9657, -363.5375) -> (-339.9671, -363.5375)
  line L1134 (-334.4679, -354.0125) -> (-339.9671, -344.4875)
  line L1135 (-339.9671, -363.5375) -> (-334.4679, -354.0125)
  line L1136 (-320.7197, -333.375) -> (-331.7182, -333.375)
  line L1137 (-331.7182, -333.375) -> (-337.2175, -342.9)
  line L1138 (-337.2175, -342.9) -> (-331.7182, -352.425)
  line L1139 (-331.7182, -352.425) -> (-320.7197, -352.425)
  line L1140 (-315.2205, -342.9) -> (-320.7197, -333.375)
  line L1141 (-320.7197, -352.425) -> (-315.2205, -342.9)
  line L1142 (-301.4723, -322.2625) -> (-312.4708, -322.2625)
  line L1143 (-312.4708, -322.2625) -> (-317.9701, -331.7875)
  line L1144 (-317.9701, -331.7875) -> (-312.4708, -341.3125)
  line L1145 (-312.4708, -341.3125) -> (-301.4723, -341.3125)
  line L1146 (-295.973, -331.7875) -> (-301.4723, -322.2625)
  line L1147 (-301.4723, -341.3125) -> (-295.973, -331.7875)
  line L1148 (-282.2249, -311.15) -> (-293.2234, -311.15)
  line L1149 (-293.2234, -311.15) -> (-298.7227, -320.675)
  line L1150 (-298.7227, -320.675) -> (-293.2234, -330.2)
  line L1151 (-293.2234, -330.2) -> (-282.2249, -330.2)
  line L1152 (-276.7256, -320.675) -> (-282.2249, -311.15)
  line L1153 (-282.2249, -330.2) -> (-276.7256, -320.675)
  line L1154 (-262.9775, -300.0375) -> (-273.976, -300.0375)
  line L1155 (-273.976, -300.0375) -> (-279.4753, -309.5625)
  line L1156 (-279.4753, -309.5625) -> (-273.976, -319.0875)
  line L1157 (-273.976, -319.0875) -> (-262.9775, -319.0875)
  line L1158 (-257.4782, -309.5625) -> (-262.9775, -300.0375)
  line L1159 (-262.9775, -319.0875) -> (-257.4782, -309.5625)
  line L1160 (-243.7301, -288.925) -> (-254.7286, -288.925)
  line L1161 (-254.7286, -288.925) -> (-260.2278, -298.45)
  line L1162 (-260.2278, -298.45) -> (-254.7286, -307.975)
  line L1163 (-254.7286, -307.975) -> (-243.7301, -307.975)
  line L1164 (-238.2308, -298.45) -> (-243.7301, -288.925)
  line L1165 (-243.7301, -307.975) -> (-238.2308, -298.45)
  line L1166 (-224.4826, -277.8125) -> (-235.4812, -277.8125)
  line L1167 (-235.4812, -277.8125) -> (-240.9804, -287.3375)
  line L1168 (-240.9804, -287.3375) -> (-235.4812, -296.8625)
  line L1169 (-235.4812, -296.8625) -> (-224.4826, -296.8625)
  line L1170 (-218.9834, -287.3375) -> (-224.4826, -277.8125)
  line L1171 (-224.4826, -296.8625) -> (-218.9834, -287.3375)
  line L1172 (-205.2352, -266.7) -> (-216.2337, -266.7)
  line L1173 (-216.2337, -266.7) -> (-221.733, -276.225)
  line L1174 (-221.733, -276.225) -> (-216.2337, -285.75)
  line L1175 (-216.2337, -285.75) -> (-205.2352, -285.75)
  line L1176 (-199.736, -276.225) -> (-205.2352, -266.7)
  line L1177 (-205.2352, -285.75) -> (-199.736, -276.225)
  line L1178 (-185.9878, -255.5875) -> (-196.9863, -255.5875)
  line L1179 (-196.9863, -255.5875) -> (-202.4856, -265.1125)
  line L1180 (-202.4856, -265.1125) -> (-196.9863, -274.6375)
  line L1181 (-196.9863, -274.6375) -> (-185.9878, -274.6375)
  line L1182 (-180.4886, -265.1125) -> (-185.9878, -255.5875)
  line L1183 (-185.9878, -274.6375) -> (-180.4886, -265.1125)
  line L1184 (-166.7404, -244.475) -> (-177.7389, -244.475)
  line L1185 (-177.7389, -244.475) -> (-183.2382, -254)
  line L1186 (-183.2382, -254) -> (-177.7389, -263.525)
  line L1187 (-177.7389, -263.525) -> (-166.7404, -263.525)
  line L1188 (-161.2411, -254) -> (-166.7404, -244.475)
  line L1189 (-166.7404, -263.525) -> (-161.2411, -254)
  line L1190 (-147.493, -233.3625) -> (-158.4915, -233.3625)
  line L1191 (-158.4915, -233.3625) -> (-163.9908, -242.8875)
  line L1192 (-163.9908, -242.8875) -> (-158.4915, -252.4125)
  line L1193 (-158.4915, -252.4125) -> (-147.493, -252.4125)
  line L1194 (-141.9937, -242.8875) -> (-147.493, -233.3625)
  line L1195 (-147.493, -252.4125) -> (-141.9937, -242.8875)
  line L1196 (-128.2456, -222.25) -> (-139.2441, -222.25)
  line L1197 (-139.2441, -222.25) -> (-144.7434, -231.775)
  line L1198 (-144.7434, -231.775) -> (-139.2441, -241.3)
  line L1199 (-139.2441, -241.3) -> (-128.2456, -241.3)
  line L1200 (-122.7463, -231.775) -> (-128.2456, -222.25)
  line L1201 (-128.2456, -241.3) -> (-122.7463, -231.775)
  line L1202 (-108.9982, -211.1375) -> (-119.9967, -211.1375)
  line L1203 (-119.9967, -211.1375) -> (-125.4959, -220.6625)
  line L1204 (-125.4959, -220.6625) -> (-119.9967, -230.1875)
  line L1205 (-119.9967, -230.1875) -> (-108.9982, -230.1875)
  line L1206 (-103.4989, -220.6625) -> (-108.9982, -211.1375)
  line L1207 (-108.9982, -230.1875) -> (-103.4989, -220.6625)
  line L1208 (-89.7507, -200.025) -> (-100.7493, -200.025)
  line L1209 (-100.7493, -200.025) -> (-106.2485, -209.55)
  line L1210 (-106.2485, -209.55) -> (-100.7493, -219.075)
  line L1211 (-100.7493, -219.075) -> (-89.7507, -219.075)
  line L1212 (-84.2515, -209.55) -> (-89.7507, -200.025)
  line L1213 (-89.7507, -219.075) -> (-84.2515, -209.55)
  line L1214 (-70.5033, -188.9125) -> (-81.5018, -188.9125)
  line L1215 (-81.5018, -188.9125) -> (-87.0011, -198.4375)
  line L1216 (-87.0011, -198.4375) -> (-81.5018, -207.9625)
  line L1217 (-81.5018, -207.9625) -> (-70.5033, -207.9625)
  line L1218 (-65.0041, -198.4375) -> (-70.5033, -188.9125)
  line L1219 (-70.5033, -207.9625) -> (-65.0041, -198.4375)
  line L1220 (-51.2559, -177.8) -> (-62.2544, -177.8)
  line L1221 (-62.2544, -177.8) -> (-67.7537, -187.325)
  line L1222 (-67.7537, -187.325) -> (-62.2544, -196.85)
  line L1223 (-62.2544, -196.85) -> (-51.2559, -196.85)
  line L1224 (-45.7566, -187.325) -> (-51.2559, -177.8)
  line L1225 (-51.2559, -196.85) -> (-45.7566, -187.325)
  line L1226 (-32.0085, -166.6875) -> (-43.007, -166.6875)
  line L1227 (-43.007, -166.6875) -> (-48.5063, -176.2125)
  line L1228 (-48.5063, -176.2125) -> (-43.007, -185.7375)
  line L1229 (-43.007, -185.7375) -> (-32.0085, -185.7375)
  line L1230 (-26.5092, -176.2125) -> (-32.0085, -166.6875)
  line L1231 (-32.0085, -185.7375) -> (-26.5092, -176.2125)
  line L1232 (-12.7611, -155.575) -> (-23.7596, -155.575)
  line L1233 (-23.7596, -155.575) -> (-29.2589, -165.1)
  line L1234 (-29.2589, -165.1) -> (-23.7596, -174.625)
  line L1235 (-23.7596, -174.625) -> (-12.7611, -174.625)
  line L1236 (-7.2618, -165.1) -> (-12.7611, -155.575)
  line L1237 (-12.7611, -174.625) -> (-7.2618, -165.1)
  line L1238 (6.4863, -144.4625) -> (-4.5122, -144.4625)
  line L1239 (-4.5122, -144.4625) -> (-10.0114, -153.9875)
  line L1240 (-10.0114, -153.9875) -> (-4.5122, -163.5125)
  line L1241 (-4.5122, -163.5125) -> (6.4863, -163.5125)